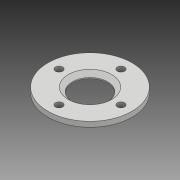
# Autodesk Inventor part: bar2
Saved by Autodesk Inventor 2018 (Build 220112000, 112)
## iProperties
Created: 2019-02-22
Part Number: bar2
Material: 一般
Document SubType Name: Modeling
Designer: ku_sk
Density: 1 g/cm^3
Appearance: 既定
Author: ku_sk
## iProperties of the stored document bar2_3D プリント.ipt
Created: 2019-02-22
Part Number: bar2_3D プリント
Material: 一般
Document SubType Name: Modeling
Designer: ku_sk
Density: 1 g/cm^3
Appearance: 既定
Author: ku_sk
Autodesk Inventor part; units mm, degrees
ref_plane "YZ Plane" through (0, 0, 0) normal (1, 0, 0) x (0, 1, 0)
ref_plane "XZ Plane" through (0, 0, 0) normal (0, 1, 0) x (-1, 0, 0)
ref_plane "XY Plane" through (0, 0, 0) normal (0, 0, 1) x (1, 0, 0)
sketch "スケッチ1" plane through (0, 0, 0) normal (0, 0, 1) x (1, 0, 0)
  circle A0 centre (0, 0) radius 20.35
  circle A1 centre (0, 0) radius 8.5
  dimension "d0" = 40.7
  dimension "d1" = 17
  constraints: 2 centre point, 2 coincident
  measures "d0" diameter of A0
  measures "d1" diameter of A1
extrude "押し出し1" add sketch "スケッチ1" along normal blind 2.5
sketch "スケッチ2" plane through (0, 0, 0) normal (0, 0, -1) x (-1, 0, 0)
  circle A0 centre (0, 15) radius 1.75
  line L0 (0, -28.49) -> (0, 28.49) projected
  point P0 (0, 0)
  dimension "d4" = 15
  dimension "d5" = 3.5
  constraints: 1 centre point, 1 point on line
  measures "d4" distance of point (0, 0) A0.centre
  measures "d5" diameter of A0
extrude "押し出し2" cut sketch "スケッチ2" against normal blind 5
pattern_circular "円形状パターン1" count 4 over 360 about axis through (0, 0, -10) along (0, 0, 1) of "押し出し2"
chamfer "面取り1" distance 2 angle 45 1 edges at (-8.5, 0, 2.5)
